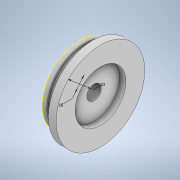
# Autodesk Inventor part: Крышка_пром_новая
Saved by Autodesk Inventor 2021 (Build 250183000, 183)
## iProperties
Created: 2023-04-26
Part Number: Крышка_пром_новая
Material: Типовые
Document SubType Name: Modeling
Designer: gdevc
Density: 1 g/cm^3
Appearance: По умолчанию
Mass: 25.9991 g
Surface Area: 93.9755 cm^2
Volume: 25.9991 cm^3
Author: gdevc
Autodesk Inventor part; units mm, degrees
ref_plane "YZ Plane" through (0, 0, 0) normal (1, 0, 0) x (0, 1, 0)
ref_plane "XZ Plane" through (0, 0, 0) normal (0, 1, 0) x (-1, 0, 0)
ref_plane "XY Plane" through (0, 0, 0) normal (0, 0, 1) x (1, 0, 0)
sketch "Эскиз1" plane through (0, 0, 0) normal (0, 0, 1) x (1, 0, 0)
  line L0 (0, 0) -> (0, 26)
  line L1 (9, 26.1456) -> (9, 30.5)
  line L2 (9, 30.5) -> (14.45, 30.5)
  line L3 (14.45, 30.5) -> (14.45, 17.5)
  line L4 (14.45, 17.5) -> (10, 17.5)
  line L5 (10, 17.5) -> (10, 0)
  line L6 (10, 0) -> (0, 0)
  line L7 (0, 26) -> (3.5, 26)
  line L8 (3.5, 26) -> (4, 25.5)
  line L9 (4, 25.5) -> (9, 25.5)
  line L10 (9, 25.5) -> (9, 26.1456)
  dimension "d1" = 52
  dimension "d2" = 0.5
  dimension "d3" = 45
  dimension "d4" = 5
  dimension "d5" = 14.45
  dimension "d6" = 10
  dimension "d7" = 35
  dimension "d8" = 4.5
  dimension "d23" = 9
  constraints: 22 end point, 6 perpendicular, 1 horizontal, 1 parallel, 1 vertical
  measures "d1" diameter of L7 L6
  measures "d2" distance between parallel lines of L7 L9
  measures "d3" angle of L7 L8
  measures "d4" distance of L8.end L9.end
  measures "d5" distance between parallel lines of L3 L0
  measures "d6" distance between parallel lines of L0 L5
  measures "d7" diameter of L4 L6
  measures "d8" distance between parallel lines of L7 L2
  measures "d23" distance between parallel lines of L0 L1
revolve "Вращение1" add sketch "Эскиз1" angle 360 about axis through (10, 0, 0) along (-1, 0, 0)
sketch "Эскиз2" plane through (0, 0, 0) normal (-1, 0, 0) x (0, 0, 1)
  circle A0 centre (0, 0) radius 26 projected
  circle A1 centre (0, 0) radius 10
  circle A2 centre (0, 0) radius 5
  point P0 (0, 0)
  dimension "d10" = 20
  dimension "d11" = 10
  constraints: 2 centre point, 2 coincident
  measures "d10" diameter of A1
  measures "d11" diameter of A2
extrude "Выдавливание1" cut sketch "Эскиз2" against normal through all contours A2
fillet "Сопряжение2" radius 0.5 1 edges at (4, -25.5, 0)
chamfer "Фаска2" distance 1 angle 45 1 edges at (0, 0, -5)
thread "Резьба3" size "M10x0.5" class "6H" standard "ANSI Metric M Profile" length 10
